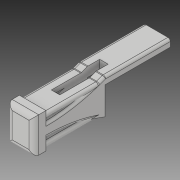
# Autodesk Inventor part: pushbar
Saved by Autodesk Inventor 2018 (Build 220112000, 112)
## iProperties
Created: 2019-02-21
Part Number: pushbar
Material: 一般
Document SubType Name: Modeling
Designer: ku_sk
Density: 1 g/cm^3
Appearance: 既定
Author: ku_sk
## iProperties of the stored document pushbar_3D プリント.ipt
Created: 2019-02-22
Part Number: pushbar_3D プリント
Material: 一般
Document SubType Name: Modeling
Designer: ku_sk
Density: 1 g/cm^3
Appearance: 既定
Author: ku_sk
Autodesk Inventor part; units mm, degrees
ref_plane "YZ Plane" through (0, 0, 0) normal (1, 0, 0) x (0, 1, 0)
ref_plane "XZ Plane" through (0, 0, 0) normal (0, 1, 0) x (-1, 0, 0)
ref_plane "XY Plane" through (0, 0, 0) normal (0, 0, 1) x (1, 0, 0)
sketch "スケッチ1" plane through (0, 0, 0) normal (1, 0, 0) x (0, 1, 0)
  line L0 (-5.5, 7.25) -> (5.5, 7.25)
  line L1 (5.5, 7.25) -> (5.5, -7.25)
  line L2 (5.5, -7.25) -> (-5.5, -7.25)
  line L3 (-5.5, -7.25) -> (-5.5, 7.25)
  line L4 (-7.7, 0) -> (7.7, 0) projected
  line L5 (0, -10.15) -> (0, 10.15) projected
  point P0 (0, 0)
  point P1 (5.5, 0)
  point P2 (0, 7.25)
  dimension "d0" = 14.5
  dimension "d1" = 11
  constraints: 8 end point, 2 midpoint, 2 parallel, 2 point on line, 1 horizontal, 1 perpendicular
  measures "d0" distance of L0.end L1.end
  measures "d1" distance of L0.start L0.end
extrude "押し出し1" add sketch "スケッチ1" along normal mid plane 37.5
sketch "スケッチ2" plane through (-18.75, 5.5, 7.25) normal (0, 1, 0) x (1, 0, 0)
  line L0 (0, 0) -> (0, 14.5) projected
  line L1 (0, 14.5) -> (33, 14.5)
  line L2 (33, 14.5) -> (33, 4)
  line L3 (33, 4) -> (0, 4)
  line L4 (0, 4) -> (0, 14.5)
  point P0 (18.75, 7.25)
  dimension "d4" = 33
  dimension "d5" = 10.5
  constraints: 8 end point, 2 parallel, 1 horizontal, 1 perpendicular
  measures "d4" distance of L2.end L3.end
  measures "d5" distance of L1.end L2.end
extrude "押し出し2" cut sketch "スケッチ2" against normal through all
sketch "スケッチ4" plane through (18.75, 0, 0) normal (1, 0, 0) x (0, 0, -1)
  line L0 (7.25, 5.5) -> (-7.25, 5.5) projected
  line L1 (-7.25, 5.5) -> (-7.25, -5.5) projected
  line L2 (-7.25, -5.5) -> (7.25, -5.5) projected
  line L3 (7.25, -5.5) -> (7.25, 5.5) projected
  point P0 (0, 0)
extrude "押し出し4" add sketch "スケッチ4" along normal blind 25
sketch "スケッチ5" plane through (-18.75, -5.5, 3.25) normal (0, -1, 0) x (1, 0, 0)
  line L0 (33, -10.5) -> (62.5, -10.5) projected
  line L1 (33, -10.5) -> (33, 0) projected
  arc A0 (57.5, -5.8194) -> (33, -10.5) centre (57.5, -72.2801) ccw
  line L2 (0, 4) -> (62.5, 4) projected
  arc A1 (33, 4) -> (57.5, -0.6806) centre (57.5, 65.7801) ccw
  line L3 (0, 4) -> (62.5, 4) projected
  line L4 (33, 0) -> (33, -10.5) projected
  line L5 (57.5, -5.8194) -> (57.5, -10.5)
  line L6 (57.5, -0.6806) -> (57.5, 4)
  line L7 (62.5, 4) -> (62.5, -10.5) projected
  point P0 (18.75, -3.25)
  point P1 (45.0284, 0.5)
  point P2 (45.0284, -7)
  dimension "d16" = 3.5
  dimension "d17" = 3.5
  dimension "d20" = 5
  constraints: 6 point on circle, 4 end point, 4 point on line, 2 centre point, 2 collinear, 2 line through centre, 1 perpendicular
  measures "d16" distance from line of L2 point (45.028, 0.5)
  measures "d17" distance from line of L0 point (45.028, -7)
  measures "d20" distance between parallel lines of L7 L6
extrude "押し出し6" cut sketch "スケッチ5" against normal up to surface (11 mm away)
sketch "スケッチ6" plane through (-18.75, -5.5, 3.25) normal (0, -1, 0) x (1, 0, 0)
  line L0 (57.5, 3) -> (35.6897, 3)
  line L1 (35.6897, 3) -> (35.6897, 1)
  line L2 (35.6897, 1) -> (57.5, 1)
  line L3 (57.5, 1) -> (57.5, 3)
  line L4 (57.5, -7.5) -> (35.6897, -7.5)
  line L5 (35.6897, -7.5) -> (35.6897, -9.5)
  line L6 (35.6897, -9.5) -> (57.5, -9.5)
  line L7 (57.5, -9.5) -> (57.5, -7.5)
  line L8 (57.5, 4) -> (62.5, 4) projected
  line L9 (57.5, -10.5) -> (62.5, -10.5) projected
  line L10 (57.5, 4) -> (57.5, -0.6806) projected
  arc A0 (33, 4) -> (57.5, -0.6806) centre (57.5, 65.7801) ccw projected
  point P0 (18.75, -3.25)
  dimension "d23" = 2
  dimension "d24" = 1
  dimension "d25" = 2
  dimension "d26" = 1
  constraints: 16 end point, 4 parallel, 2 horizontal, 2 perpendicular, 2 point on line, 1 collinear, 1 point on circle
  measures "d23" distance of L2.end L0.start
  measures "d24" distance between parallel lines of L8 L0
  measures "d25" distance of L6.end L4.start
  measures "d26" distance between parallel lines of L9 L6
extrude "押し出し7" add sketch "スケッチ6" against normal up to surface (11 mm away) contours L3 L2 A0 L0 | A0 L2 L1 | L7 L6 L5 L4
fillet "フィレット1" radius 1 18 edges at (31.2768, -5.5, 2.9908) (31.3242, -5.5, 4.25) (31.2768, -5.5, -2.9908) (31.3242, -5.5, -4.25) (31.3242, 5.5, 4.25) (31.2768, 5.5, 2.9908) (31.2768, 5.5, -2.9908) (31.3242, 5.5, -4.25) (27.8448, -5.5, 6.25) (27.8448, -5.5, -6.25) (27.8448, 5.5, 6.25) (27.8448, 5.5, -6.25) (-2.25, -5.5, 7.25) (-2.25, 5.5, 7.25) (15.5894, 5.5, 6.7355) (15.5894, -5.5, 6.7355) (14.25, 0, 7.25) (16.9397, 0, 6.25)
chamfer "面取り2" distance 1 angle 45 2 edges at (-2.25, -5.5, 3.25) (-2.25, 5.5, 3.25)
sketch "スケッチ8" plane through (-18.75, 4.5, 7.25) normal (0, 0, 1) x (1, 0, 0)
  line L0 (33, -9) -> (33, -10) projected
  line L1 (33, 0) -> (33, -9) projected
  line L2 (33, 1) -> (33, 0) projected
  line L3 (33, -10) -> (33, 1) projected
  line L4 (28, -6.25) -> (48, -6.25)
  line L5 (48, -6.25) -> (48, -2.75)
  line L6 (48, -2.75) -> (28, -2.75)
  line L7 (28, -2.75) -> (28, -6.25)
  line L8 (48, -4.5) -> (28, -4.5)
  point P0 (18.75, -4.5)
  point P1 (33, -4.5)
  dimension "d33" = 3.5
  dimension "d34" = 5
  dimension "d35" = 20
  constraints: 10 end point, 3 midpoint, 2 parallel, 1 horizontal, 1 perpendicular, 1 point on line
  measures "d33" distance of L4.end L5.end
  measures "d34" distance between parallel lines of L1 L7
  measures "d35" distance of L5.end L6.end
extrude "押し出し8" cut sketch "スケッチ8" against normal blind 12
fillet "フィレット2" radius 2 4 edges at (43.75, 0, 7.25) (43.75, -5.5, 0) (43.75, 5.5, 0) (43.75, 0, -7.25)
sketch "スケッチ9" plane through (-18.75, 0, 0) normal (-1, 0, 0) x (0, 0, 1)
  line L0 (3.25, 4.5) -> (4.25, 5.5) projected
  line L1 (3.25, 4.5) -> (3.25, -4.5) projected
  line L2 (4.25, -5.5) -> (3.25, -4.5) projected
  line L3 (4.25, -5.5) -> (6.25, -5.5) projected
  arc A0 (6.25, -5.5) -> (7.25, -4.5) centre (6.25, -4.5) ccw projected
  line L4 (7.25, -4.5) -> (7.25, 4.5) projected
  arc A1 (7.25, 4.5) -> (6.25, 5.5) centre (6.25, 4.5) ccw projected
  line L5 (6.25, 5.5) -> (4.25, 5.5) projected
  point P0 (0, 0)
extrude "押し出し9" cut sketch "スケッチ9" against normal blind 5
chamfer "面取り3" distance 1 angle 45 6 edges at (-13.75, 5.2071, 6.9571) (-13.75, 0, 7.25) (-13.75, -5.2071, 6.9571) (-13.75, -5.5, 5.25) (-13.75, 5.5, 5.25) (-13.75, 0, 3.25)
equation "\"d17\" = d16"
equation "\"d25\" = d23"
equation "\"d26\" = d24"
